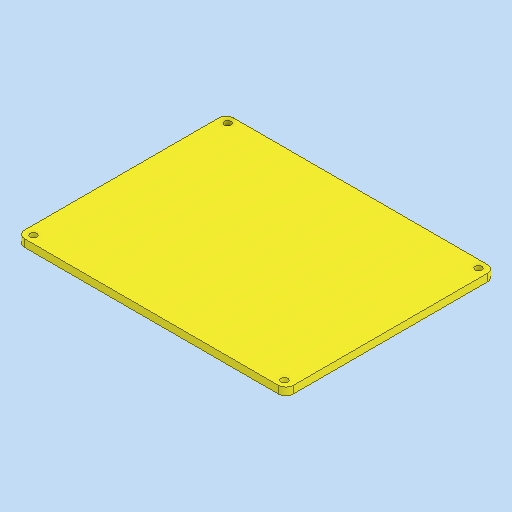
# Autodesk Inventor part: крышка акб
Saved by Autodesk Inventor 2025 (Build 290162000, 162)
## iProperties
Created: 2025-02-26
Part Number: крышка акб
Material: Пластик АБС
Document SubType Name: Modeling
Designer: volko
Density: 1.06 g/cm^3
Appearance: Канареечный
Mass: 133.109 g
Surface Area: 536.697 cm^2
Volume: 125.575 cm^3
Author: volko
Autodesk Inventor part; units mm, degrees
ref_plane "YZ Plane" through (0, 0, 0) normal (1, 0, 0) x (0, 1, 0)
ref_plane "XZ Plane" through (0, 0, 0) normal (0, 1, 0) x (-1, 0, 0)
ref_plane "XY Plane" through (0, 0, 0) normal (0, 0, 1) x (1, 0, 0)
sketch "Эскиз1" plane through (0, 0, 0) normal (0, 1, 0) x (-1, 0, 0)
  line L0 (90, 70) -> (-90, 70)
  line L1 (-90, 70) -> (-90, -70)
  line L2 (-90, -70) -> (90, -70)
  line L3 (90, -70) -> (90, 70)
  line L4 (-126, 0) -> (126, 0) projected
  line L5 (0, -98) -> (0, 98) projected
  point P0 (0, 0)
  dimension "d1" = 180
  dimension "d2" = 140
  constraints: 8 end point, 2 parallel, 1 horizontal, 1 perpendicular, 2 other
  measures "d1" distance of L0.start L0.end
  measures "d2" distance of L2.end L0.start
extrude "Выдавливание1" add sketch "Эскиз1" along normal blind 5
fillet "Сопряжение1" radius 5 4 edges at (90, 2.5, -70) (90, 2.5, 70) (-90, 2.5, 70) (-90, 2.5, -70)
sketch "Эскиз2" plane through (0, 5, 0) normal (0, 1, 0) x (1, 0, 0)
  line L0 (0, 98) -> (0, -98) projected
  line L1 (-126, 0) -> (126, 0) projected
  line L2 (-90, 65) -> (-90, -65) projected
  line L3 (-85, -70) -> (85, -70) projected
  point P0 (0, 0)
  point P1 (-84, -65)
  point P2 (-84, 65)
  point P3 (84, -65)
  point P4 (84, 65)
  dimension "d15" = 130
  dimension "d18" = 168
  dimension "d21" = 6
  dimension "d22" = 5
  constraints: 1 horizontal, 1 vertical, 3 other
  measures "d15" distance of point (-84, -65) point (-84, 65)
  measures "d18" distance of point (-84, -65) point (84, -65)
  measures "d21" distance from line of L2 point (-84, -65)
  measures "d22" distance from line of point (-84, -65) L3
hole "Отверстие1" at (-84, 5, 65) at (84, 5, 65) at (-84, 5, -65) at (84, 5, -65) direction (0, -1, 0) diameter 4.5 end through all
